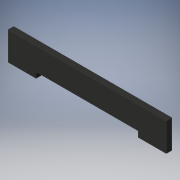
# Autodesk Inventor part: EBF_003.1-front-plate_cup-holder
Saved by Autodesk Inventor 2019 (Build 230136000, 136)
## iProperties
Created: 2019-02-28
Part Number: EBF_003.1-front-plate_cup-holder
Material: Generic
Document SubType Name: Modeling
Designer: Rene
Density: 1 g/cm^3
Appearance: Rubber - Black
Author: Rene
Autodesk Inventor part; units mm, degrees
ref_plane "YZ Plane" through (0, 0, 0) normal (1, 0, 0) x (0, 1, 0)
ref_plane "XZ Plane" through (0, 0, 0) normal (0, 1, 0) x (-1, 0, 0)
ref_plane "XY Plane" through (0, 0, 0) normal (0, 0, 1) x (1, 0, 0)
sketch "Sketch1" plane through (0, 0, 0) normal (0, 0, 1) x (1, 0, 0)
  line L0 (-70, -10) -> (70, -10)
  line L1 (70, -10) -> (70, 10)
  line L2 (70, 10) -> (-70, 10)
  line L3 (-70, 10) -> (-70, -10)
  point P0 (0, 0)
  dimension "width" = 140
  dimension "d1" = 70
  dimension "d2" = 20
  dimension "d3" = 10
  constraints: 8 end point, 2 parallel, 1 horizontal, 1 perpendicular
  measures "width" distance of L0.start L0.end
  measures "d1" horizontal distance of point (0, 0) L0.start
  measures "d2" distance of L2.end L0.start
  measures "d3" vertical distance of point (0, 0) L0.start
extrude "Extrusion1" add sketch "Sketch1" along normal blind 5
sketch "Sketch4" plane through (-70, -10, 0) normal (0, -1, 0) x (1, 0, 0)
  line L0 (0, 0) -> (140, 0) projected
  line L1 (0, 5) -> (140, 5) projected
  line L2 (0, 0) -> (24.8, 0)
  line L3 (24.8, 0) -> (24.8, 5)
  line L4 (24.8, 5) -> (0, 5)
  line L5 (0, 5) -> (0, 0)
  point P0 (70, 0)
  dimension "d28" = 24.8
  constraints: 8 end point, 2 parallel, 1 horizontal, 1 perpendicular, 1 point on line
  measures "d28" distance from line of L0.start L3
extrude "Extrusion4" add sketch "Sketch4" along normal blind 5
mirror "Mirror1" about plane through (0, 0, 0) normal (1, 0, 0) of "Extrusion4"
equation "\"d1\" = 0.5 * width"
equation "\"d3\" = 0.5 * d2"
body "Solid1"
